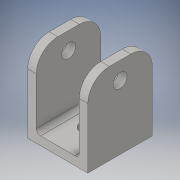
# Autodesk Inventor part: linear actuator bracket
Saved by Autodesk Inventor 2016 (Build 200138000, 138)
## iProperties
Created: 2016-03-07
Part Number: linear actuator bracket
Material: Generic
Document SubType Name: Modeling
Designer: tyler
Density: 1 g/cm^3
Appearance: Default
Author: tyler
Autodesk Inventor part; units mm, degrees
ref_plane "YZ Plane" through (0, 0, 0) normal (1, 0, 0) x (0, 1, 0)
ref_plane "XZ Plane" through (0, 0, 0) normal (0, 1, 0) x (-1, 0, 0)
ref_plane "XY Plane" through (0, 0, 0) normal (0, 0, 1) x (1, 0, 0)
sketch "Sketch1" plane through (0, 0, 0) normal (0, 0, 1) x (1, 0, 0)
  line L0 (-11.8297, 9.3175) -> (-7.8297, 9.3175)
  line L1 (-7.8297, 9.3175) -> (-7.8297, -24.6825)
  line L2 (-11.8297, -24.6825) -> (-11.8297, 9.3175)
  line L3 (16.1703, -24.6825) -> (16.1703, -28.6825)
  line L4 (16.1703, -28.6825) -> (-11.8297, -28.6825)
  line L5 (-11.8297, -28.6825) -> (-11.8297, -24.6825)
  line L6 (12.1703, -24.6825) -> (12.1703, 9.3175)
  line L7 (12.1703, 9.3175) -> (16.1703, 9.3175)
  line L8 (16.1703, 9.3175) -> (16.1703, -24.6825)
  line L9 (12.1703, -24.6825) -> (-7.8297, -24.6825)
  point P0 (0, 0)
  dimension "d0" = 4
  dimension "d1" = 34
  dimension "d5" = 4
  dimension "d6" = 4
  dimension "d7" = 34
  dimension "d14" = 24
  dimension "d15" = 28
  dimension "d16" = 38
  dimension "d18" = 9.3175
  constraints: 20 end point, 7 parallel, 2 horizontal, 1 perpendicular
  measures "d0" distance of L1.end L2.start
  measures "d1" distance of L0.end L1.end
  measures "d5" distance of L3.start L3.end
  measures "d6" distance of L6.end L7.end
  measures "d7" distance of L6.start L6.end
  measures "d14" distance between parallel lines of L3 L1
  measures "d15" distance between parallel lines of L3 L2
  measures "d16" distance between parallel lines of L7 L4
  measures "d18" distance from line of point (0, 0) L7
extrude "Extrusion1" add sketch "Sketch1" along normal blind 30
sketch "Sketch2" plane through (-11.8297, -28.6825, 0) normal (-1, 0, 0) x (0, 0, 1)
  line L0 (0, 0) -> (0, 38) construction
  line L1 (0, 0) -> (30, 0) construction
  line L2 (30, 38) -> (30, 0) construction
  line L3 (0, 38) -> (30, 38) construction
  line L4 (0, 38) -> (30, 38) construction
  line L5 (15, 38) -> (15, 0) construction
  circle A0 centre (15, 29.8727) radius 3.25
  point P0 (0, 28.6825)
  dimension "d10" = 6.5
  constraints: 2 end point, 2 midpoint, 1 centre point, 1 point on line
  measures "d10" diameter of A0
extrude "Extrusion2" cut sketch "Sketch2" against normal through all
fillet "Fillet1" radius 10 4 edges at (-9.8297, 9.3175, 0) (14.1703, 9.3175, 0) (-9.8297, 9.3175, 30) (14.1703, 9.3175, 30)
sketch "Sketch3" plane through (-7.8297, -24.6825, 0) normal (0, 1, 0) x (1, 0, 0)
  line L0 (0, 0) -> (20, 0) projected
  line L1 (0, 0) -> (0, -30) projected
  line L2 (20, -30) -> (0, -30) projected
  line L3 (20, 0) -> (20, -30) projected
  circle A0 centre (10, -15) radius 4.25
  point P0 (7.8297, 0)
  dimension "d19" = 8.5
  constraints: 1 centre point
  measures "d19" diameter of A0
extrude "Extrusion3" cut sketch "Sketch3" against normal through all contours A0
fillet "Fillet2" radius 2 2 edges at (-7.8297, -24.6825, 15) (12.1703, -24.6825, 15)
equation "\"d1\" = d7"
body "Solid1"
